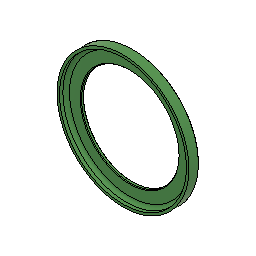
Distinctive Ring v5 (Autodesk Fusion 360 design; units mm, degrees)
Autodesk Fusion 360 part; units mm, degrees
sketch "Sketch1" plane through (0, 0, 0) normal (0, 0, 1) x (1, 0, 0)
  circle A0 centre (0, 0) radius 14.6
  circle A1 centre (0, 0) radius 19
  circle A2 centre (0, 0) radius 19.75
  dimension "d1" = 29.2
  dimension "d2" = 38
  dimension "d3" = 39.5
  constraint coincident A0.centre A1.centre
  constraint concentric A1 A2
  measures "d1" diameter of A0
  measures "d2" diameter of A1
  measures "d3" diameter of A2
extrude "Extrude3" add sketch "Sketch1" along normal blind 1 contours A1
extrude "Extrude4" add sketch "Sketch1" along normal blind 3 contours A2
fillet "Fillet1" radius 1 1 edges at (-17.7142, -6.8707, 1)
chamfer "Chamfer1" distance 0.2 angle 45 1 edges at (-18.4135, -7.1419, 0)
chamfer "Chamfer2" distance 0.2 angle 45 2 edges at (-13.612, 5.2796, 1) (-13.612, 5.2796, 0)
extrude "Extrude1" [suppressed]
extrude "Extrude2" [suppressed]
named bodies: "Distinctive Ring", "Distinctive ring"
